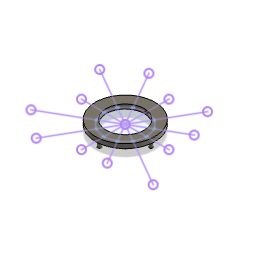
top_frame v1 (Autodesk Fusion 360 design; units mm, degrees)
Autodesk Fusion 360 part; units mm, degrees
note: some values were not read from the file. Set by a fixed rule: which sketch regions a step uses; which face or edge a step refers to.
sketch "스케치1" plane through (0, 0, 0) normal (0, 1, 0) x (1, 0, 0)
  circle A0 centre (0, 0) radius 28 construction
  circle A1 centre (0, 0) radius 43
  circle A2 centre (0, 0) radius 68
  circle A3 centre (0, 0) radius 48 construction
  line L0 (-100, 0) -> (100, 0) construction
  line L1 (0, 100) -> (0, -100) construction
  line L2 (-136.6025, -78.8675) -> (100, 57.735) construction
  line L3 (-137.8994, 79.6163) -> (151.432, -87.4293) construction
  line L4 (-74.5024, -129.042) -> (68.9117, 119.3585) construction
  line L5 (-74.0212, 128.2085) -> (56.0866, -97.1449) construction
  circle A4 centre (0, 0) radius 63 construction
  line L6 (-59.5273, -59.5273) -> (58.6358, 58.6358) construction
  line L7 (-67.2013, 67.2013) -> (116.9721, -116.9721) construction
  dimension "d1" = 56
  dimension "d2" = 15
  dimension "d3" = 25
  dimension "d5" = 5
  dimension "d8" = 30
  dimension "d10" = 30
  dimension "d11" = 60
  dimension "d12" = 60
  dimension "d39" = 5
  dimension "d55" = 45
  dimension "d56" = 45
  constraint coincident A0.centre A1.centre
  constraint concentric A0 A1
  constraint concentric A2 A3
  constraint horizontal L0
  constraint vertical L1
  constraint coincident A0.centre L2
  constraint coincident A0.centre L3
  constraint coincident A0.centre L4
  constraint coincident A0.centre L5
  constraint concentric A2 A4
  constraint coincident A0.centre L6
  constraint coincident A0.centre L7
  measures "d1" diameter of A0
  measures "d2" distance of A0 A1
  measures "d3" distance of A1 A2
  measures "d5" distance of A1 A3
  measures "d8" angle of L0 L2
  measures "d10" angle of L0 L3
  measures "d11" angle of L0 L4
  measures "d12" angle of L0 L5
  measures "d39" distance of A2 A4
  measures "d55" angle of L0 L6
  measures "d56" angle of L0 L7
sketch "스케치2" plane through (0, 0, 0) normal (0, 1, 0) x (1, 0, 0)
  line L0 (-2.25, 49.8) -> (2.25, 49.8)
  line L1 (2.25, 49.8) -> (2.25, 48)
  line L2 (2.25, 48) -> (-2.25, 48)
  line L3 (-2.25, 48) -> (-2.25, 49.8)
  line L4 (-2.25, 48) -> (2.25, 49.8) construction
  line L5 (2.25, 48) -> (-2.25, 49.8) construction
  line L6 (0, 48) -> (0, 49.8) construction
  line L7 (-48, -2.25) -> (-49.8, -2.25)
  line L8 (-49.8, -2.25) -> (-48, 2.25) construction
  line L9 (-48, 2.25) -> (-48, -2.25)
  line L10 (-49.8, 0) -> (-48, 0) construction
  line L11 (-49.8, -2.25) -> (-49.8, 2.25)
  line L12 (-49.8, 2.25) -> (-48, -2.25) construction
  line L13 (-49.8, 2.25) -> (-48, 2.25)
  circle A0 centre (0, 0) radius 48
  line L14 (-22.9514, 44.2531) -> (-22.0514, 42.6942)
  line L15 (-26.8486, 42.0031) -> (-22.9514, 44.2531)
  line L16 (-22.0514, 42.6942) -> (-25.9486, 40.4442)
  line L17 (-25.9486, 40.4442) -> (-22.9514, 44.2531) construction
  line L18 (-25.9486, 40.4442) -> (-26.8486, 42.0031)
  line L19 (-22.0514, 42.6942) -> (-26.8486, 42.0031) construction
  line L20 (-24, 41.5692) -> (-24.9, 43.1281) construction
  line L21 (-74.0212, 128.2085) -> (56.0866, -97.1449)
  line L22 (-44.2531, 22.9514) -> (-42.0031, 26.8486)
  line L23 (-42.6942, 22.0514) -> (-42.0031, 26.8486) construction
  line L24 (-40.4442, 25.9486) -> (-44.2531, 22.9514) construction
  line L25 (-42.6942, 22.0514) -> (-44.2531, 22.9514)
  line L26 (-42.0031, 26.8486) -> (-40.4442, 25.9486)
  line L27 (-40.4442, 25.9486) -> (-42.6942, 22.0514)
  line L28 (-41.5692, 24) -> (-43.1281, 24.9) construction
  line L29 (-137.8994, 79.6163) -> (151.432, -87.4293)
  line L30 (-100, 0) -> (100, 0)
  line L31 (-44.2531, -22.9514) -> (-40.4442, -25.9486) construction
  line L32 (-43.1281, -24.9) -> (-41.5692, -24) construction
  line L33 (-40.4442, -25.9486) -> (-42.0031, -26.8486)
  line L34 (-44.2531, -22.9514) -> (-42.6942, -22.0514)
  line L35 (-42.0031, -26.8486) -> (-42.6942, -22.0514) construction
  line L36 (-42.0031, -26.8486) -> (-44.2531, -22.9514)
  line L37 (-42.6942, -22.0514) -> (-40.4442, -25.9486)
  line L38 (-26.8486, -42.0031) -> (-22.0514, -42.6942) construction
  line L39 (-24.9, -43.1281) -> (-24, -41.5692) construction
  line L40 (-22.0514, -42.6942) -> (-22.9514, -44.2531)
  line L41 (-26.8486, -42.0031) -> (-25.9486, -40.4442)
  line L42 (-22.9514, -44.2531) -> (-25.9486, -40.4442) construction
  line L43 (-22.9514, -44.2531) -> (-26.8486, -42.0031)
  line L44 (-25.9486, -40.4442) -> (-22.0514, -42.6942)
  line L45 (0, -49.8) -> (0, -48) construction
  line L46 (2.25, -48) -> (2.25, -49.8)
  line L47 (2.25, -49.8) -> (-2.25, -48) construction
  line L48 (-2.25, -49.8) -> (2.25, -48) construction
  line L49 (-2.25, -48) -> (2.25, -48)
  line L50 (-2.25, -49.8) -> (-2.25, -48)
  line L51 (2.25, -49.8) -> (-2.25, -49.8)
  line L52 (24.9, -43.1281) -> (24, -41.5692) construction
  line L53 (25.9486, -40.4442) -> (26.8486, -42.0031)
  line L54 (26.8486, -42.0031) -> (22.0514, -42.6942) construction
  line L55 (22.9514, -44.2531) -> (25.9486, -40.4442) construction
  line L56 (22.0514, -42.6942) -> (25.9486, -40.4442)
  line L57 (22.9514, -44.2531) -> (22.0514, -42.6942)
  line L58 (26.8486, -42.0031) -> (22.9514, -44.2531)
  line L59 (43.1281, -24.9) -> (41.5692, -24) construction
  line L60 (42.6942, -22.0514) -> (44.2531, -22.9514)
  line L61 (44.2531, -22.9514) -> (40.4442, -25.9486) construction
  line L62 (42.0031, -26.8486) -> (42.6942, -22.0514) construction
  line L63 (40.4442, -25.9486) -> (42.6942, -22.0514)
  line L64 (42.0031, -26.8486) -> (40.4442, -25.9486)
  line L65 (44.2531, -22.9514) -> (42.0031, -26.8486)
  line L66 (48, 0) -> (49.8, 0) construction
  line L67 (49.8, -2.25) -> (48, -2.25)
  line L68 (48, -2.25) -> (49.8, 2.25) construction
  line L69 (48, 2.25) -> (49.8, -2.25) construction
  line L70 (49.8, 2.25) -> (49.8, -2.25)
  line L71 (48, 2.25) -> (49.8, 2.25)
  line L72 (48, -2.25) -> (48, 2.25)
  line L73 (41.5692, 24) -> (43.1281, 24.9) construction
  line L74 (44.2531, 22.9514) -> (42.6942, 22.0514)
  line L75 (42.6942, 22.0514) -> (42.0031, 26.8486) construction
  line L76 (40.4442, 25.9486) -> (44.2531, 22.9514) construction
  line L77 (42.0031, 26.8486) -> (44.2531, 22.9514)
  line L78 (40.4442, 25.9486) -> (42.0031, 26.8486)
  line L79 (42.6942, 22.0514) -> (40.4442, 25.9486)
  line L80 (24, 41.5692) -> (24.9, 43.1281) construction
  line L81 (26.8486, 42.0031) -> (25.9486, 40.4442)
  line L82 (25.9486, 40.4442) -> (22.9514, 44.2531) construction
  line L83 (22.0514, 42.6942) -> (26.8486, 42.0031) construction
  line L84 (22.9514, 44.2531) -> (26.8486, 42.0031)
  line L85 (22.0514, 42.6942) -> (22.9514, 44.2531)
  line L86 (25.9486, 40.4442) -> (22.0514, 42.6942)
  line L87 (-136.6025, -78.8675) -> (100, 57.735)
  line L88 (-74.5024, -129.042) -> (68.9117, 119.3585)
  line L89 (0, 100) -> (0, -100)
  dimension "d13" = 4.5
  dimension "d14" = 1.8
  constraint horizontal L0
  constraint vertical L1
  constraint horizontal L2
  constraint vertical L3
  constraint midpoint L2 L6.start
  constraint midpoint L0 L6.end
  constraint midpoint L10.start L11
  constraint midpoint L10.end L9
  constraint midpoint L20.start L16
  constraint midpoint L20.end L15
  constraint perpendicular L16 L18
  constraint perpendicular L14 L16
  constraint perpendicular L14 L15
  constraint collinear L20 L21
  constraint perpendicular L11 L13
  constraint perpendicular L7 L11
  constraint perpendicular L7 L9
  constraint midpoint L28.start L27
  constraint midpoint L28.end L22
  constraint perpendicular L25 L27
  constraint perpendicular L26 L27
  constraint perpendicular L22 L26
  constraint collinear L28 L29
  constraint collinear L10 L30
  constraint midpoint L32.start L36
  constraint midpoint L32.end L37
  constraint perpendicular L34 L36
  constraint perpendicular L33 L36
  constraint perpendicular L33 L37
  constraint midpoint L39.start L43
  constraint midpoint L39.end L44
  constraint perpendicular L41 L43
  constraint perpendicular L40 L43
  constraint perpendicular L40 L44
  constraint midpoint L45.start L51
  constraint midpoint L45.end L49
  constraint perpendicular L50 L51
  constraint perpendicular L46 L51
  constraint perpendicular L46 L49
  constraint midpoint L52.start L58
  constraint midpoint L52.end L56
  constraint perpendicular L57 L58
  constraint perpendicular L53 L58
  constraint perpendicular L53 L56
  constraint midpoint L59.start L65
  constraint midpoint L59.end L63
  constraint perpendicular L64 L65
  constraint perpendicular L60 L65
  constraint perpendicular L60 L63
  constraint midpoint L66.start L72
  constraint midpoint L66.end L70
  constraint perpendicular L71 L72
  constraint perpendicular L67 L72
  constraint perpendicular L67 L70
  constraint midpoint L73.start L79
  constraint midpoint L73.end L77
  constraint perpendicular L78 L79
  constraint perpendicular L74 L79
  constraint perpendicular L74 L77
  constraint midpoint L80.start L86
  constraint midpoint L80.end L84
  constraint perpendicular L85 L86
  constraint perpendicular L81 L86
  constraint perpendicular L81 L84
  constraint collinear L32 L87
  constraint collinear L39 L88
  constraint collinear L45 L89
  constraint collinear L21 L52
  constraint collinear L29 L59
  constraint collinear L30 L66
  constraint collinear L73 L87
  constraint collinear L80 L88
  constraint equal L3 L14
  constraint equal L0 L15
  constraint equal L18 L26
  constraint equal L15 L22
  constraint equal L13 L25
  constraint equal L11 L22
  constraint equal L11 L36
  constraint equal L7 L34
  constraint equal L33 L41
  constraint equal L36 L43
  constraint equal L40 L50
  constraint equal L43 L51
  constraint equal L46 L57
  constraint equal L51 L58
  constraint equal L53 L64
  constraint equal L58 L65
  constraint equal L60 L67
  constraint equal L65 L70
  constraint equal L71 L74
  constraint equal L70 L77
  constraint equal L78 L81
  constraint equal L77 L84
  constraint collinear L6 L89
  constraint tangent A0 L63
  constraint tangent A0 L56
  constraint tangent A0 L49
  constraint tangent A0 L44
  constraint tangent A0 L37
  constraint tangent L9 A0
  constraint tangent A0 L27
  constraint tangent A0 L16
  constraint tangent L2 A0
  constraint tangent A0 L86
  constraint tangent A0 L79
  constraint tangent A0 L72
  measures "d13" distance of L0.start L0.end
  measures "d14" distance of L0.start L2.end
sketch "스케치3" plane through (0, 0, 0) normal (0, 1, 0) x (1, 0, 0)
  circle A0 centre (59, 0) radius 4
  circle A1 centre (0, 0) radius 63
  line L0 (-100, 0) -> (100, 0)
  circle A2 centre (0, 59) radius 4
  line L1 (0, 100) -> (0, -100)
  circle A3 centre (-59, 0) radius 4
  circle A4 centre (0, -59) radius 4
  circle A5 centre (42.78, -42.78) radius 2.5
  line L2 (-67.2013, 67.2013) -> (116.9721, -116.9721)
  circle A6 centre (-42.78, -42.78) radius 2.5
  line L3 (-59.5273, -59.5273) -> (58.6358, 58.6358)
  circle A7 centre (-42.78, 42.78) radius 2.5
  circle A8 centre (42.78, 42.78) radius 2.5
  dimension "d40" = 8
  dimension "d57" = 5
  constraint tangent A0 A1
  constraint coincident A0.centre L0
  constraint tangent A1 A2
  constraint coincident A2.centre L1
  constraint tangent A1 A3
  constraint coincident L0 A3.centre
  constraint tangent A1 A4
  constraint coincident L1 A4.centre
  constraint equal A0 A2
  constraint equal A2 A3
  constraint equal A3 A4
  constraint coincident A5.centre L2
  constraint tangent A1 A5
  constraint coincident A6.centre L3
  constraint equal A5 A6
  constraint tangent A1 A6
  constraint equal A5 A7
  constraint coincident L2 A7.centre
  constraint tangent A1 A7
  constraint coincident L3 A8.centre
  constraint equal A5 A8
  constraint tangent A1 A8
  measures "d40" diameter of A0
  measures "d57" diameter of A5
extrude "돌출1" add sketch "스케치1" along normal blind 10
extrude "돌출2" cut sketch "스케치2" along normal blind 5 contours L84 L85 L86 L88 | L81 L84 L86 L88 | L77 L78 L79 L87 | L74 L77 L79 L87 | L30 L70 L71 L72 | L30 L67 L70 L72 | L29 L60 L63 L65 | L29 L63 L64 L65 | L21 L53 L56 L58 | L21 L56 L57 L58 | L46 L49 L51 L89 | L49 L50 L51 L89 | L40 L43 L44 L88 | L41 L43 L44 L88 | L33 L36 L37 L87 | L34 L36 L37 L87 | L7 L9 L11 L30 | L9 L11 L13 L30 | L22 L25 L27 L29 | L22 L26 L27 L29 | L15 L16 L18 L21 | L14 L15 L16 L21 | L0 L2 L3 L89 | L0 L1 L2 L89
extrude "돌출3" add sketch "스케치3" against normal blind 10 contours A0 L0 | A0 L0 | A2 L1 | A2 L1 | L1 A4 | L1 A4 | L0 A3 | L0 A3
extrude "돌출4" add 4 faces at (-60.2298, -10, 0.1987) (0.0996, -10, -57.8473) (0.0996, -10, 60.1527) (57.7702, -10, 0.1987) along direction (0, -1, 0) blind 4
extrude "돌출5" add 4 faces at (-60.2298, -14, 0.1987) (0.0996, -14, 60.1527) (0.0996, -14, -57.8473) (57.7702, -14, 0.1987) along direction (0, -1, 0) blind 3
extrude "돌출6" add sketch "스케치3" against normal blind 4 contours L3 A8 | L3 A8 | A5 L2 | A5 L2 | L2 A7 | L2 A7 | A6 L3 | A6 L3
fillet "모깎기1" radius 2 4 faces at (0.0996, -17, 60.1527) (-60.2298, -17, 0.1987) (0.0996, -17, -57.8473) (57.7702, -17, 0.1987)
